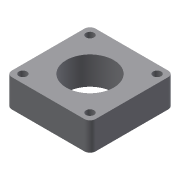
# Autodesk Inventor part: 00_fan_30mm_24mm
Saved by Autodesk Inventor 2019.4 (Build 234330000, 330)
## iProperties
Created: 2021-08-23
Part Number: 00_fan_30mm_24mm
Material: Generic
Document SubType Name: Modeling
Designer: diederichbenedict
Density: 1 g/cm^3
Appearance: Default
Author: diederichbenedict
Autodesk Inventor part; units mm, degrees
ref_plane "YZ Plane" through (0, 0, 0) normal (1, 0, 0) x (0, 1, 0)
ref_plane "XZ Plane" through (0, 0, 0) normal (0, 1, 0) x (-1, 0, 0)
ref_plane "XY Plane" through (0, 0, 0) normal (0, 0, 1) x (1, 0, 0)
sketch "Sketch1" plane through (0, 0, 0) normal (0, 1, 0) x (-1, 0, 0)
  line L0 (15, -15) -> (-15, -15)
  line L1 (-15, -15) -> (-15, 15)
  line L2 (-15, 15) -> (15, 15)
  line L3 (15, 15) -> (15, -15)
  line L4 (15, -15) -> (-15, 15) construction
  line L5 (-15, -15) -> (15, 15) construction
  point P0 (0, 0)
  dimension "d0" = 30
  dimension "d1" = 30
  constraints: 12 end point, 2 midpoint, 2 parallel, 1 horizontal, 1 perpendicular
  measures "d0" distance of L1.end L2.end
  measures "d1" distance of L0.end L1.end
extrude "Extrusion1" add sketch "Sketch1" along normal blind 10
sketch "Sketch2" plane through (0, 0, 0) normal (0, -1, 0) x (1, 0, 0)
  line L0 (12, 12) -> (-12, 12) construction
  line L1 (-12, 12) -> (-12, -12) construction
  line L2 (-12, -12) -> (12, -12) construction
  line L3 (12, -12) -> (12, 12) construction
  line L4 (12, 12) -> (-12, -12) construction
  line L5 (-12, 12) -> (12, -12) construction
  circle A0 centre (12, 12) radius 1.45
  circle A1 centre (12, -12) radius 1.45
  circle A2 centre (-12, -12) radius 1.45
  circle A3 centre (-12, 12) radius 1.45
  circle A4 centre (0, 0) radius 13.5
  circle A5 centre (0, 0) radius 8.5
  dimension "d4" = 24
  dimension "d5" = 24
  dimension "d6" = 2.9
  dimension "d7" = 2.9
  dimension "d8" = 2.9
  dimension "d9" = 2.9
  dimension "d10" = 27
  dimension "d11" = 17
  constraints: 12 end point, 6 centre point, 6 coincident, 2 midpoint, 2 parallel, 1 horizontal, 1 perpendicular
  measures "d4" distance of L2.end L1.end
  measures "d5" distance of L1.end L0.end
  measures "d6" diameter of A0
  measures "d7" diameter of A1
  measures "d8" diameter of A2
  measures "d9" diameter of A3
  measures "d10" diameter of A4
  measures "d11" diameter of A5
extrude "Extrusion2" cut sketch "Sketch2" against normal through all
fillet "Fillet1" radius 2 4 edges at (15, 5, 15) (-15, 5, 15) (15, 5, -15) (-15, 5, -15)
ref_plane "Work Plane1" through (13, 0, 0) normal (0, 0, -1) x (-1, 0, 0)
ref_plane "Work Plane2" through (0, 0, 13) normal (1, 0, 0) x (0, 0, -1)
body "Solid1"
